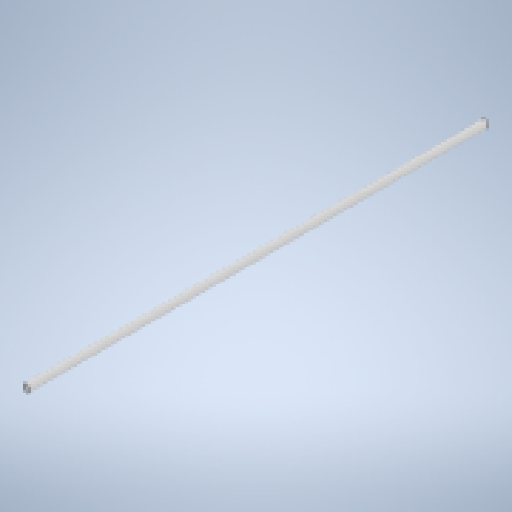
# Autodesk Inventor part: ось колес2
Saved by Autodesk Inventor 2023.1 (Build 271208000, 208)
## iProperties
Created: 2024-12-17
Part Number: ось колес2
Material: Типовые
Document SubType Name: Modeling
Designer: DELL
Density: 1 g/cm^3
Appearance: По умолчанию
Author: DELL
Autodesk Inventor part; units mm, degrees
ref_plane "YZ Plane" through (0, 0, 0) normal (1, 0, 0) x (0, 1, 0)
ref_plane "XZ Plane" through (0, 0, 0) normal (0, 1, 0) x (-1, 0, 0)
ref_plane "XY Plane" through (0, 0, 0) normal (0, 0, 1) x (1, 0, 0)
ref_plane "РабПлоскость1" through (-33.1795, -18.2761, -5.1998) normal (0, 0, 1) x (0.9782133, 0.2076025, 0)
ref_plane "РабПлоскость2" through (-33.1795, -18.2761, -5.1998) normal (0, 0, 1) x (0.9782133, 0.2076025, 0)
sketch "Эскиз1" plane through (0, 0, 0) normal (0, 0, 1) x (1, 0, 0)
  circle A0 centre (0, 0) radius 2.5
  dimension "d0" = 5
  constraints: 1 centre point, 1 coincident
  measures "d0" diameter of A0
extrude "Выдавливание1" add sketch "Эскиз1" against normal up to surface (5.1998 mm away)
sketch "Эскиз2" plane through (0, 0, 0) normal (0, 0, 1) x (1, 0, 0)
  circle A0 centre (0, 0) radius 2.5
  constraints: 1 centre point, 1 coincident
ref_plane "РабПлоскость3" through (-19.9176, -17.3177, 300) normal (0, 0, 1) x (0.9879927, -0.1545007, 0)
extrude "Выдавливание2" add sketch "Эскиз2" along normal up to surface (300 mm away)
